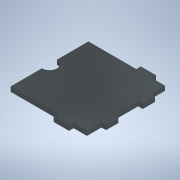
# Autodesk Inventor part: SoporteCircuito
Saved by Autodesk Inventor 2020.2 (Build 242310000, 310)
## iProperties
Created: 2020-03-18
Part Number: SoporteCircuito
Material: Iron, Cast
Document SubType Name: Modeling
Designer: ARQ SEVILLA R
Density: 7.15 g/cm^3
Appearance: Iron Gray
Author: ARQ SEVILLA R
Autodesk Inventor part; units mm, degrees
ref_plane "YZ Plane" through (0, 0, 0) normal (1, 0, 0) x (0, 1, 0)
ref_plane "XZ Plane" through (0, 0, 0) normal (0, 1, 0) x (-1, 0, 0)
sketch "Sketch1" plane through (0, 0, 0) normal (0, 1, 0) x (-1, 0, 0)
  line L0 (53, -54) -> (53, -3)
  line L1 (21.75, 0) -> (11.75, 0)
  line L2 (3, -3) -> (3, -12.5)
  line L3 (3, -12.5) -> (0, -12.5)
  line L4 (0, -12.5) -> (0, -20.5)
  line L5 (0, -20.5) -> (3, -20.5)
  line L6 (0, -28.5) -> (26.5, -28.5) construction
  line L7 (26.5, -28.5) -> (26.5, -57) construction
  line L8 (3, -20.5) -> (3, -28.5)
  line L9 (3, -54) -> (3, -44.5)
  line L10 (3, -44.5) -> (0, -44.5)
  line L11 (0, -44.5) -> (0, -36.5)
  line L12 (0, -36.5) -> (3, -36.5)
  line L13 (3, -36.5) -> (3, -28.5)
  line L14 (3, -3) -> (11.75, -3)
  line L15 (11.75, -3) -> (11.75, 0)
  line L16 (11.75, 0) -> (21.75, 0)
  line L17 (21.75, 0) -> (21.75, -3)
  line L18 (21.75, -3) -> (53, -3)
  line L19 (21.75, -57) -> (11.75, -57)
  line L20 (3, -54) -> (11.75, -54)
  line L21 (11.75, -54) -> (11.75, -57)
  line L22 (21.75, -57) -> (21.75, -54)
  line L23 (21.75, -54) -> (53, -54)
  point P0 (0, 0)
  dimension "d4" = 8
  dimension "d6" = 8.75
  dimension "d7" = 10
  constraints: 48 end point, 10 symmetric about line, 5 perpendicular, 1 parallel, 1 point on line, 1 vertical
  measures "d4" distance of L3.end L4.end
  measures "d6" distance of L2.start L14.end
  measures "d7" distance of L1.start L1.end
extrude "Extrusion1" add sketch "Sketch1" along normal blind 3
sketch "Sketch2" plane through (0, 0, 0) normal (0, -1, 0) x (1, 0, 0)
  line L0 (-53, -54) -> (-53, -3) projected
  arc A0 (-53, -33.5) -> (-53, -23.5) centre (-53, -28.5) ccw
  line L1 (-53, -33.5) -> (-53, -23.5)
  point P0 (0, 0)
  dimension "d10" = 10
  constraints: 2 end point, 2 point on circle, 2 point on line, 1 centre point, 1 collinear, 1 midpoint
  measures "d10" diameter of A0
ref_plane "Work Plane1" through (-57, 11.25, -57) normal (0, 1, 0) x (0, 0, 1)
extrude "Extrusion2" cut sketch "Sketch2" against normal up to surface (11.25 mm away)
body "Solid1"
